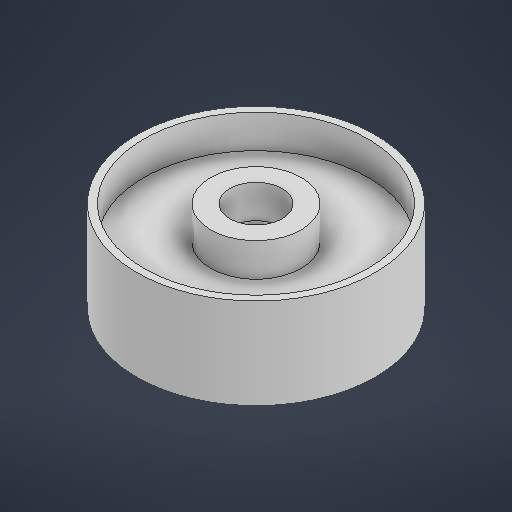
# Autodesk Inventor part: Wheel
Saved by Autodesk Inventor 2026 (Build 300175000, 175)
## iProperties
Created: 2025-05-07
Part Number: Wheel
Material: Generic
Document SubType Name: Modeling
Designer: Ritul Kumari
Density: 1 g/cm^3
Appearance: Default
Author: Ritul Kumari
Autodesk Inventor part; units mm, degrees
ref_plane "YZ Plane" through (0, 0, 0) normal (1, 0, 0) x (0, 1, 0)
ref_plane "XZ Plane" through (0, 0, 0) normal (0, 1, 0) x (-1, 0, 0)
ref_plane "XY Plane" through (0, 0, 0) normal (0, 0, 1) x (1, 0, 0)
sketch "Sketch1" plane through (0, 0, 0) normal (0, 0, 1) x (1, 0, 0)
  line L0 (0, 0) -> (279.4, 0)
  line L1 (279.4, 0) -> (279.4, 355.6)
  line L2 (279.4, 355.6) -> (482.6, 355.6)
  line L3 (482.6, 355.6) -> (482.6, 0)
  line L4 (482.6, 0) -> (1193.8, 0)
  line L5 (1193.8, 0) -> (1193.8, 355.6)
  line L6 (1193.8, 355.6) -> (1270, 355.6)
  line L7 (1270, 355.6) -> (1270, 0)
  line L8 (1270, 0) -> (1270, -609.6)
  line L9 (1270, 0) -> (1879.6, 0) construction
  line L10 (1270, -609.6) -> (1193.8, -609.6)
  line L11 (1193.8, -609.6) -> (1193.8, -254)
  line L12 (1193.8, -254) -> (482.6, -254)
  line L13 (482.6, -254) -> (482.6, -609.6)
  line L14 (482.6, -609.6) -> (279.4, -609.6)
  line L15 (279.4, -609.6) -> (279.4, -254)
  line L16 (279.4, -254) -> (0, -254)
  line L17 (0, -254) -> (0, 0)
  dimension "d0" = 279.4
  dimension "d1" = 355.6
  dimension "d2" = 203.2
  dimension "d3" = 711.2
  dimension "d4" = 355.6
  dimension "d5" = 76.2
  dimension "d6" = 609.6
  dimension "d7" = 90
  dimension "d8" = 76.2
  dimension "d9" = 355.6
  dimension "d10" = 355.6
  dimension "d11" = 203.2
  dimension "d12" = 355.6
  constraints: 36 end point, 9 perpendicular, 6 horizontal, 3 vertical, 1 point on line
  measures "d0" distance of L0.start L0.end
  measures "d1" distance of L0.end L1.end
  measures "d2" distance of L1.end L2.end
  measures "d3" distance of L3.end L4.end
  measures "d4" distance of L4.end L5.end
  measures "d5" distance of L5.end L6.end
  measures "d6" distance of L7.end L8.end
  measures "d7" angle of L8 L9
  measures "d8" distance of L8.end L10.end
  measures "d9" distance of L10.end L11.end
  measures "d10" distance of L12.end L13.end
  measures "d11" distance of L13.end L14.end
  measures "d12" distance of L14.end L15.end
revolve "Revolution1" add sketch "Sketch1" angle 360 about axis through (0, -254, 0) along (0, 1, 0)
